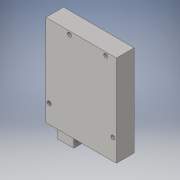
# Autodesk Inventor part: arduino uno
Saved by Autodesk Inventor 2016 (Build 200138000, 138)
## iProperties
Created: 2017-09-13
Part Number: arduino uno
Material: Generic
Document SubType Name: Modeling
Designer: student
Density: 1 g/cm^3
Appearance: Default
Author: student
Autodesk Inventor part; units mm, degrees
ref_plane "YZ Plane" through (0, 0, 0) normal (1, 0, 0) x (0, 1, 0)
ref_plane "XZ Plane" through (0, 0, 0) normal (0, 1, 0) x (-1, 0, 0)
ref_plane "XY Plane" through (0, 0, 0) normal (0, 0, 1) x (1, 0, 0)
sketch "Sketch1" plane through (0, 0, 0) normal (0, 0, 1) x (1, 0, 0)
  line L0 (-26.6827, 34.4805) -> (26.6827, 34.4805)
  line L1 (26.6827, 34.4805) -> (26.6827, -34.4805)
  line L2 (26.6827, -34.4805) -> (-26.6827, -34.4805)
  line L3 (-26.6827, -34.4805) -> (-26.6827, 34.4805)
  circle A0 centre (24.0919, -18.8595) radius 1.5113
  circle A1 centre (-24.0919, -20.5105) radius 1.5113
  circle A2 centre (-8.7503, 32.0675) radius 1.5113
  circle A3 centre (18.6563, 32.0675) radius 1.5113
  point P0 (0, 0)
  dimension "d0" = 53.3654
  dimension "d1" = 68.961
  dimension "d2" = 3.0226
  dimension "d3" = 3.0226
  dimension "d4" = 15.621
  dimension "d5" = 13.97
  dimension "d6" = 2.5908
  dimension "d7" = 2.5908
  dimension "d8" = 3.0226
  dimension "d9" = 3.0226
  dimension "d11" = 17.9324
  dimension "d12" = 8.0264
  dimension "d13" = 2.413
  constraints: 8 end point, 4 centre point, 2 parallel, 1 horizontal, 1 horizontal alignment, 1 perpendicular
  measures "d0" distance of L1.end L2.end
  measures "d1" distance of L1.end L0.end
  measures "d2" diameter of A0
  measures "d3" diameter of A1
  measures "d4" distance from line of L2 A0.centre
  measures "d5" distance from line of L2 A1.centre
  measures "d6" distance from line of L1 A0.centre
  measures "d7" distance from line of L3 A1.centre
  measures "d8" diameter of A2
  measures "d9" diameter of A3
  measures "d11" distance from line of A2.centre L3
  measures "d12" distance from line of L1 A3.centre
  measures "d13" distance from line of L0 A2.centre
extrude "Extrusion1" add sketch "Sketch1" along normal blind 13.4112
sketch "Sketch2" plane through (-26.6827, -34.4805, 0) normal (0, -1, 0) x (1, 0, 0)
  line L0 (0, 0) -> (53.3654, 0) projected
  line L1 (8.9662, 13.4061) -> (21.082, 13.4061)
  line L2 (21.082, 13.4061) -> (21.082, 2.6111)
  line L3 (21.082, 2.6111) -> (8.9662, 2.6111)
  line L4 (8.9662, 2.6111) -> (8.9662, 13.4061)
  line L5 (8.9662, 13.4061) -> (21.082, 2.6111) construction
  line L6 (21.082, 13.4061) -> (8.9662, 2.6111) construction
  line L7 (0, 0) -> (0, 13.4112) projected
  point P0 (26.6827, 0)
  point P1 (15.0241, 8.0086)
  dimension "d16" = 12.1158
  dimension "d17" = 10.795
  dimension "d18" = 8.9662
  constraints: 12 end point, 2 midpoint, 2 parallel, 1 horizontal, 1 perpendicular
  measures "d16" distance of L2.end L3.end
  measures "d17" distance of L2.end L1.end
  measures "d18" distance between parallel lines of L7 L4
extrude "Extrusion2" add sketch "Sketch2" along normal blind 6.2992
body "Solid1"
